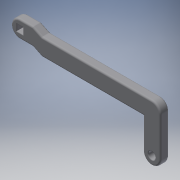
# Autodesk Inventor part: Lift Arm Lower
Saved by Autodesk Inventor 2017 (Build 210142000, 142)
## iProperties
Created: 2015-06-06
Part Number: Lift Arm Lower
Material: Generic
Document SubType Name: Modeling
Designer: Dale
Density: 1 g/cm^3
Appearance: Default
Author: Dale
## iProperties of the stored document Lift Arm Lower_3DPrint.ipt
Created: 2017-08-20
Part Number: Lift Arm Lower_3DPrint
Material: Generic
Document SubType Name: Modeling
Designer: Dale
Density: 1 g/cm^3
Appearance: Default
Author: Dale
Autodesk Inventor part; units mm, degrees
ref_plane "YZ Plane" through (0, 0, 0) normal (1, 0, 0) x (0, 1, 0)
ref_plane "XZ Plane" through (0, 0, 0) normal (0, 1, 0) x (-1, 0, 0)
ref_plane "XY Plane" through (0, 0, 0) normal (0, 0, 1) x (1, 0, 0)
sketch "Sketch4" plane through (0, 0, 0) normal (0, 0, 1) x (1, 0, 0)
  line L0 (1.3586, -0.1628) -> (1.3586, 19.8372)
  line L1 (1.3586, 19.8372) -> (26.3586, 19.8372)
  line L2 (26.3586, 19.8372) -> (36.8586, 14.8372)
  line L3 (36.8586, 14.8372) -> (173.3586, 14.8372)
  line L4 (173.3586, 14.8372) -> (173.3586, -50.1628)
  line L5 (173.3586, -50.1628) -> (153.3586, -50.1628)
  line L6 (153.3586, -50.1628) -> (153.3586, -5.1628)
  line L7 (153.3586, -5.1628) -> (36.8586, -5.1628)
  line L8 (36.8586, -5.1628) -> (26.3586, -0.1628)
  line L9 (26.3586, -0.1628) -> (1.3586, -0.1628)
  dimension "d55" = 20
  dimension "d56" = 25
  dimension "d57" = 5
  dimension "d58" = 20
  dimension "d59" = 45
  dimension "d60" = 152
  dimension "d61" = 10.5
  constraints: 20 end point, 5 parallel, 3 perpendicular, 2 vertical, 1 point on line, 1 vertical alignment
  measures "d55" distance of L0.start L0.end
  measures "d56" distance of L0.end L1.end
  measures "d57" distance between parallel lines of L9 L7
  measures "d58" distance of L4.end L5.end
  measures "d59" distance of L5.end L6.end
  measures "d60" distance between parallel lines of L6 L0
  measures "d61" horizontal distance of L2.end L1.end
extrude "Arm Base" add sketch "Sketch4" along normal blind 10
sketch "Sketch5" plane through (0, 0, 10) normal (0, 0, 1) x (1, 0, 0)
  line L0 (153.3586, -50.1628) -> (173.3586, -50.1628) projected
  line L1 (153.3586, -5.1628) -> (153.3586, -50.1628) projected
  point P0 (163.3586, -40.1628)
  dimension "d62" = 10
  dimension "d63" = 10
  measures "d62" distance from line of L0 point (163.359, -40.163)
  measures "d63" distance from line of L1 point (163.359, -40.163)
hole "Pivot Holes" at (163.3586, -40.1628, 10) direction (0, 0, -1) diameter 8 end through all
sketch "Sketch6" plane through (0, 0, 10) normal (0, 0, 1) x (1, 0, 0)
  line L0 (7.8586, 13.3372) -> (14.8586, 13.3372)
  line L1 (14.8586, 13.3372) -> (14.8586, 6.3372)
  line L2 (14.8586, 6.3372) -> (7.8586, 6.3372)
  line L3 (7.8586, 6.3372) -> (7.8586, 13.3372)
  line L4 (1.3586, 19.8372) -> (1.3586, -0.1628) projected
  point P0 (0, 0)
  point P1 (7.8586, 9.8372)
  point P2 (1.3586, 9.8372)
  dimension "d48" = 7
  dimension "d64" = 6.5
  constraints: 8 end point, 2 midpoint, 2 parallel, 2 perpendicular, 1 horizontal, 1 horizontal alignment
  measures "d48" distance of L0.start L0.end
  measures "d64" distance of point (7.859, 9.837) point (1.359, 9.837)
extrude "Extrusion5" cut sketch "Sketch6" against normal up to next
fillet "Fillet2" radius 10 5 edges at (1.3586, -0.1628, 5) (1.3586, 19.8372, 5) (173.3586, -50.1628, 5) (153.3586, -50.1628, 5) (173.3586, 14.8372, 5)
fillet "Fillet3" radius 2 26 edges at (170.4298, 11.9084, 10) (173.3586, -17.6628, 10) (170.4298, -47.234, 10) (153.3586, -22.6631, 10) (100.1089, 14.8372, 10) (95.1086, -5.1628, 10) (170.4298, -47.234, 0) (153.3586, -22.6631, 0) (170.4298, 11.9084, 0) (100.1089, 14.8372, 0) (173.3586, -17.6628, 0) (95.1086, -5.1628, 0) (18.8584, -0.1628, 0) (18.8584, 19.8372, 0) (4.2874, 2.766, 0) (18.8584, 19.8372, 10) (18.8584, -0.1628, 10) (4.2874, 2.766, 10) (31.6086, 17.3372, 10) (31.6086, -2.6628, 10) (31.6086, -2.6628, 0) (31.6086, 17.3372, 0) (26.3586, 19.8372, 5) (36.8586, 14.8372, 5) (26.3586, -0.1628, 5) (36.8586, -5.1628, 5)
fillet "Fillet4" radius 1 2 edges at (163.3586, -36.1628, 10) (163.3586, -36.1628, 0)
fillet "Fillet5" radius 1 8 edges at (7.8586, 9.8372, 10) (11.3586, 13.3372, 10) (14.8586, 9.8372, 10) (11.3586, 6.3372, 10) (7.8586, 9.8372, 0) (11.3586, 6.3372, 0) (14.8586, 9.8372, 0) (11.3586, 13.3372, 0)
body "Solid2"
